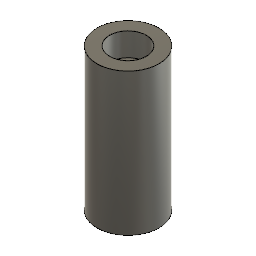
buttonhat v3 (Autodesk Fusion 360 design; units mm, degrees)
Autodesk Fusion 360 part; units mm, degrees
sketch "Sketch1" plane through (0, 0, 0) normal (0, 1, 0) x (1, 0, 0)
  circle A0 centre (0, 0) radius 3.048
  dimension "d1" = 6.096
  measures "d1" diameter of A0
extrude "Extrude1" add sketch "Sketch1" along normal blind 13.97
sketch "Sketch2" plane through (0, 13.97, 0) normal (0, 1, 0) x (-1, 0, 0)
  circle A0 centre (0, 0) radius 3.048
  circle A1 centre (0, 0) radius 1.7961
  dimension "d4" = 3.5921
  measures "d4" diameter of A1
extrude "Extrude2" cut sketch "Sketch2" against normal blind 2.286 contours A1
